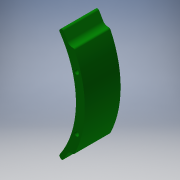
# Autodesk Inventor part: Goal
Saved by Autodesk Inventor 2016 (Build 200138000, 138)
## iProperties
Created: 2015-08-20
Part Number: Goal
Material: Generic
Document SubType Name: Modeling
Designer: TFHulbert
Density: 1 g/cm^3
Appearance: Default
Author: TFHulbert
Autodesk Inventor part; units mm, degrees
ref_plane "XZ Plane" through (0, 0, 0) normal (0, 1, 0) x (-1, 0, 0)
ref_plane "XY Plane" through (0, 0, 0) normal (0, 0, 1) x (1, 0, 0)
sketch "Sketch2" plane through (0, 0, 0) normal (0, 1, 0) x (-1, 0, 0)
  arc A0 (-3.565, 94.6695) -> (-3.565, -8.3744) centre (100.201, 43.1475) ccw
  arc A1 (10.972, -26.9746) -> (17.7694, -18.565) centre (-67.181, 43.1475) ccw
  arc A2 (17.7694, -18.565) -> (17.7741, -16.2207) centre (16.1512, -17.3895) ccw
  arc A3 (17.7741, 102.5157) -> (17.7741, -16.2207) centre (100.201, 43.1475) ccw
  arc A4 (17.7741, 102.5157) -> (17.7694, 104.8601) centre (16.1512, 103.6846) ccw
  arc A5 (17.7694, 104.8601) -> (10.972, 113.2697) centre (-67.181, 43.1475) ccw
  arc A6 (-3.565, 94.6695) -> (3.8676, 97.5325) centre (-1.6208, 100.7012) ccw
  line L0 (3.8676, 97.5325) -> (9.8686, 107.9266)
  arc A7 (13.2665, 103.6551) -> (9.8686, 107.9266) centre (-67.181, 43.1475) ccw
  arc A8 (13.2665, 103.6551) -> (13.2665, -17.36) centre (100.201, 43.1475) ccw
  arc A9 (9.8686, -21.6316) -> (13.2665, -17.36) centre (-67.181, 43.1475) ccw
  line L1 (9.8686, -21.6316) -> (3.8676, -11.2375)
  arc A10 (3.8676, -11.2375) -> (-3.565, -8.3744) centre (-1.6208, -14.4061) ccw
  line L2 (-6.3804, 13.1475) -> (-1.3804, 13.1475)
  line L3 (17.3738, -14.7626) -> (18.7645, -17.1714)
  circle A11 centre (-6.3804, 73.1475) radius 2.5
  circle A12 centre (-6.3804, 13.1475) radius 2.5
  arc A13 (-2.6208, 98.9692) -> (-1.4601, 98.7077) centre (-1.6208, 100.7012) ccw
  point P0 (0, 0)
  constraints: 25 point on circle, 14 centre point, 8 end point
extrude "Extrusion2" add sketch "Sketch2" along normal blind 40
fillet "Fillet4" radius 2 6 edges at (-9.8686, 20, 107.9266) (3.565, 20, 94.6695) (-13.2665, 20, 103.6551) (-13.2665, 20, -17.36) (-9.8686, 20, -21.6316) (3.565, 20, -8.3744)
ref_plane "Work Plane1" through (-13.25, 0, 0) normal (-1, 0, 0) x (0, -1, 0)
sketch "Sketch4" plane through (-13.25, 0, 0) normal (-1, 0, 0) x (0, -1, 0)
  line L0 (-31.9197, 26.5555) -> (-31.9197, 59.312) construction
  line L1 (-31.9197, 59.312) -> (-10.9843, 59.312) construction
  line L2 (-10.9843, 59.312) -> (-10.9843, 26.5555) construction
  line L3 (-10.9843, 26.5555) -> (-31.9197, 26.5555) construction
  line L4 (0, -20.122) -> (-40, -20.122) projected
  line L5 (-40, 105.4171) -> (-40, 106.4171) projected
  line L6 (-40, -20.122) -> (-40, 106.4171)
  line L7 (-40, -16.1771) -> (-40, 102.4722) projected
  line L8 (-40, 43.1475) -> (-4.7304, 43.1475)
  spline S0 degree 2 poles (-29.9161, 28.2102) (-29.9161, 27.8593) (-30.0521, 27.3303) (-30.1509, 27.1029) knots 0 0 0 1 2 2 2
  line L9 (-30.1509, 27.1029) -> (-30.8776, 27.1029)
  line L10 (-30.8776, 27.1029) -> (-30.8776, 27.1721)
  spline S1 degree 2 poles (-30.8776, 27.1721) (-30.6823, 27.402) (-30.4723, 27.9532) (-30.4723, 28.2127) knots 0 0 0 1 2 2 2
  spline S2 degree 2 poles (-30.4723, 28.2127) (-30.4723, 28.2794) (-30.5019, 28.4945) (-30.5316, 28.5587) knots 0 0 0 1 2 2 2
  spline S3 degree 2 poles (-30.5316, 28.5587) (-30.5662, 28.6378) (-30.6922, 28.7491) (-30.7936, 28.7491) knots 0 0 0 1 2 2 2
  spline S4 degree 2 poles (-30.7936, 28.7491) (-30.9097, 28.7491) (-31.0531, 28.5686) (-31.0852, 28.445) knots 0 0 0 1 2 2 2
  spline S5 degree 2 poles (-31.0852, 28.445) (-31.1272, 28.2893) (-31.1989, 27.9359) (-31.2533, 27.7802) knots 0 0 0 1 2 2 2
  spline S6 degree 2 poles (-31.2533, 27.7802) (-31.3769, 27.4267) (-31.7995, 27.1202) (-32.1159, 27.1202) knots 0 0 0 1 2 2 2
  spline S7 degree 2 poles (-32.1159, 27.1202) (-32.5435, 27.1202) (-33.0749, 27.8444) (-33.0749, 28.3882) knots 0 0 0 1 2 2 2
  spline S8 degree 2 poles (-33.0749, 28.3882) (-33.0749, 28.6601) (-32.9637, 29.1989) (-32.8697, 29.4115) knots 0 0 0 1 2 2 2
  line L11 (-32.8697, 29.4115) -> (-32.1727, 29.4115)
  line L12 (-32.1727, 29.4115) -> (-32.1727, 29.3447)
  spline S9 degree 2 poles (-32.1727, 29.3447) (-32.3186, 29.1742) (-32.5188, 28.6848) (-32.5188, 28.4277) knots 0 0 0 1 2 2 2
  spline S10 degree 2 poles (-32.5188, 28.4277) (-32.5188, 28.3264) (-32.4891, 28.1682) (-32.4496, 28.0792) knots 0 0 0 1 2 2 2
  spline S11 degree 2 poles (-32.4496, 28.0792) (-32.4174, 28.0076) (-32.2889, 27.9038) (-32.2098, 27.9038) knots 0 0 0 1 2 2 2
  spline S12 degree 2 poles (-32.2098, 27.9038) (-32.0912, 27.9038) (-31.9552, 28.0694) (-31.9009, 28.3066) knots 0 0 0 1 2 2 2
  spline S13 degree 2 poles (-31.9009, 28.3066) (-31.8663, 28.4599) (-31.7995, 28.7441) (-31.7427, 28.9072) knots 0 0 0 1 2 2 2
  spline S14 degree 2 poles (-31.7427, 28.9072) (-31.6265, 29.2236) (-31.2409, 29.5326) (-30.9246, 29.5326) knots 0 0 0 1 2 2 2
  spline S15 degree 2 poles (-30.9246, 29.5326) (-30.4698, 29.5326) (-29.9161, 28.8183) (-29.9161, 28.2102) knots 0 0 0 1 2 2 2
  line L13 (-29.9705, 32.4985) -> (-29.9705, 31.7323)
  line L14 (-29.9705, 31.7323) -> (-31.3225, 31.7323)
  line L15 (-31.3225, 31.7323) -> (-31.3225, 30.6918)
  line L16 (-31.3225, 30.6918) -> (-29.9705, 30.6918)
  line L17 (-29.9705, 30.6918) -> (-29.9705, 29.9256)
  line L18 (-29.9705, 29.9256) -> (-33.0205, 29.9256)
  line L19 (-33.0205, 29.9256) -> (-33.0205, 30.6918)
  line L20 (-33.0205, 30.6918) -> (-31.9033, 30.6918)
  line L21 (-31.9033, 30.6918) -> (-31.9033, 31.7323)
  line L22 (-31.9033, 31.7323) -> (-33.0205, 31.7323)
  line L23 (-33.0205, 31.7323) -> (-33.0205, 32.4985)
  line L24 (-33.0205, 32.4985) -> (-29.9705, 32.4985)
  line L25 (-32.4397, 35.1728) -> (-32.4397, 33.8925)
  line L26 (-32.4397, 33.8925) -> (-31.8638, 33.8925)
  line L27 (-31.8638, 33.8925) -> (-31.8638, 35.0715)
  line L28 (-31.8638, 35.0715) -> (-31.2829, 35.0715)
  line L29 (-31.2829, 35.0715) -> (-31.2829, 33.8925)
  line L30 (-31.2829, 33.8925) -> (-29.9705, 33.8925)
  line L31 (-29.9705, 33.8925) -> (-29.9705, 33.1313)
  line L32 (-29.9705, 33.1313) -> (-33.0205, 33.1313)
  line L33 (-33.0205, 33.1313) -> (-33.0205, 35.1728)
  line L34 (-33.0205, 35.1728) -> (-32.4397, 35.1728)
  line L35 (-29.9705, 39.6144) -> (-29.9705, 38.6826)
  line L36 (-29.9705, 38.6826) -> (-31.0902, 37.8348)
  line L37 (-31.0902, 37.8348) -> (-31.0902, 37.558)
  line L38 (-31.0902, 37.558) -> (-29.9705, 37.558)
  line L39 (-29.9705, 37.558) -> (-29.9705, 36.7967)
  line L40 (-29.9705, 36.7967) -> (-33.0205, 36.7967)
  line L41 (-33.0205, 36.7967) -> (-33.0205, 38.0226)
  spline S16 degree 2 poles (-33.0205, 38.0226) (-33.0205, 38.2772) (-32.9562, 38.6529) (-32.8574, 38.8136) knots 0 0 0 1 2 2 2
  spline S17 degree 2 poles (-32.8574, 38.8136) (-32.7536, 38.9767) (-32.4298, 39.1695) (-32.1826, 39.1695) knots 0 0 0 1 2 2 2
  spline S18 degree 2 poles (-32.1826, 39.1695) (-31.8341, 39.1695) (-31.3966, 38.8531) (-31.2681, 38.5886) knots 0 0 0 1 2 2 2
  line L42 (-31.2681, 38.5886) -> (-29.9705, 39.6144)
  spline S19 degree 2 poles (-32.0862, 38.3835) (-32.2024, 38.3835) (-32.368, 38.2945) (-32.4125, 38.1932) knots 0 0 0 1 2 2 2
  spline S20 degree 2 poles (-32.4125, 38.1932) (-32.4421, 38.1215) (-32.4594, 37.946) (-32.4594, 37.815) knots 0 0 0 1 2 2 2
  line L43 (-32.4594, 37.815) -> (-32.4594, 37.558)
  line L44 (-32.4594, 37.558) -> (-31.6389, 37.558)
  line L45 (-31.6389, 37.558) -> (-31.6389, 37.7779)
  spline S21 degree 2 poles (-31.6389, 37.7779) (-31.6389, 37.9361) (-31.6784, 38.161) (-31.7402, 38.2377) knots 0 0 0 1 2 2 2
  spline S22 degree 2 poles (-31.7402, 38.2377) (-31.7995, 38.3118) (-31.9577, 38.3835) (-32.0862, 38.3835) knots 0 0 0 1 2 2 2
  spline S23 degree 2 poles (-31.4955, 42.6174) (-30.754, 42.6174) (-29.9062, 41.8265) (-29.9062, 41.1394) knots 0 0 0 1 2 2 2
  spline S24 degree 2 poles (-29.9062, 41.1394) (-29.9062, 40.4498) (-30.7639, 39.6638) (-31.4955, 39.6638) knots 0 0 0 1 2 2 2
  spline S25 degree 2 poles (-31.4955, 39.6638) (-32.2296, 39.6638) (-33.0848, 40.4498) (-33.0848, 41.1394) knots 0 0 0 1 2 2 2
  spline S26 degree 2 poles (-33.0848, 41.1394) (-33.0848, 41.8265) (-32.2345, 42.6174) (-31.4955, 42.6174) knots 0 0 0 1 2 2 2
  spline S27 degree 2 poles (-31.4955, 41.8265) (-31.7699, 41.8265) (-32.153, 41.7153) (-32.2741, 41.6189) knots 0 0 0 1 2 2 2
  spline S28 degree 2 poles (-32.2741, 41.6189) (-32.4001, 41.5225) (-32.5089, 41.2753) (-32.5089, 41.1418) knots 0 0 0 1 2 2 2
  spline S29 degree 2 poles (-32.5089, 41.1418) (-32.5089, 41.001) (-32.4075, 40.7711) (-32.279, 40.6648) knots 0 0 0 1 2 2 2
  spline S30 degree 2 poles (-32.279, 40.6648) (-32.1604, 40.5709) (-31.7674, 40.4547) (-31.4955, 40.4547) knots 0 0 0 1 2 2 2
  spline S31 degree 2 poles (-31.4955, 40.4547) (-31.2137, 40.4547) (-30.843, 40.5659) (-30.7169, 40.6623) knots 0 0 0 1 2 2 2
  spline S32 degree 2 poles (-30.7169, 40.6623) (-30.5909, 40.7587) (-30.4821, 41.0084) (-30.4821, 41.1418) knots 0 0 0 1 2 2 2
  spline S33 degree 2 poles (-30.4821, 41.1418) (-30.4821, 41.2778) (-30.5983, 41.5299) (-30.7219, 41.6213) knots 0 0 0 1 2 2 2
  spline S34 degree 2 poles (-30.7219, 41.6213) (-30.8554, 41.7202) (-31.2088, 41.8265) (-31.4955, 41.8265) knots 0 0 0 1 2 2 2
  spline S35 degree 2 poles (-30.9048, 45.5092) (-30.6774, 45.5092) (-30.3338, 45.3362) (-30.2201, 45.1929) knots 0 0 0 1 2 2 2
  spline S36 degree 2 poles (-30.2201, 45.1929) (-30.0842, 45.0198) (-29.9705, 44.6095) (-29.9705, 44.2907) knots 0 0 0 1 2 2 2
  line L46 (-29.9705, 44.2907) -> (-29.9705, 43.0722)
  line L47 (-29.9705, 43.0722) -> (-33.0205, 43.0722)
  line L48 (-33.0205, 43.0722) -> (-33.0205, 44.1474)
  spline S37 degree 2 poles (-33.0205, 44.1474) (-33.0205, 44.4835) (-32.9686, 44.8295) (-32.887, 44.9803) knots 0 0 0 1 2 2 2
  spline S38 degree 2 poles (-32.887, 44.9803) (-32.8005, 45.1459) (-32.5039, 45.3065) (-32.3111, 45.3065) knots 0 0 0 1 2 2 2
  spline S39 degree 2 poles (-32.3111, 45.3065) (-32.0887, 45.3065) (-31.7402, 45.0841) (-31.6586, 44.8864) knots 0 0 0 1 2 2 2
  line L49 (-31.6586, 44.8864) -> (-31.6438, 44.8864)
  spline S40 degree 2 poles (-31.6438, 44.8864) (-31.5845, 45.1706) (-31.2162, 45.5092) (-30.9048, 45.5092) knots 0 0 0 1 2 2 2
  spline S41 degree 2 poles (-30.9171, 44.7183) (-31.0605, 44.7183) (-31.2212, 44.6046) (-31.2632, 44.4909) knots 0 0 0 1 2 2 2
  spline S42 degree 2 poles (-31.2632, 44.4909) (-31.2904, 44.4217) (-31.2953, 44.177) (-31.2953, 43.9743) knots 0 0 0 1 2 2 2
  line L50 (-31.2953, 43.9743) -> (-31.2953, 43.8335)
  line L51 (-31.2953, 43.8335) -> (-30.5266, 43.8335)
  line L52 (-30.5266, 43.8335) -> (-30.5266, 43.8755)
  spline S43 degree 2 poles (-30.5266, 43.8755) (-30.5266, 44.1721) (-30.534, 44.3995) (-30.5859, 44.5181) knots 0 0 0 1 2 2 2
  spline S44 degree 2 poles (-30.5859, 44.5181) (-30.6329, 44.6219) (-30.8059, 44.7183) (-30.9171, 44.7183) knots 0 0 0 1 2 2 2
  spline S45 degree 2 poles (-32.1604, 44.528) (-32.2345, 44.528) (-32.3902, 44.4514) (-32.4248, 44.3723) knots 0 0 0 1 2 2 2
  spline S46 degree 2 poles (-32.4248, 44.3723) (-32.4594, 44.2981) (-32.4644, 44.0905) (-32.4644, 43.8854) knots 0 0 0 1 2 2 2
  line L53 (-32.4644, 43.8854) -> (-32.4644, 43.8335)
  line L54 (-32.4644, 43.8335) -> (-31.8168, 43.8335)
  line L55 (-31.8168, 43.8335) -> (-31.8168, 43.9298)
  spline S47 degree 2 poles (-31.8168, 43.9298) (-31.8168, 44.1251) (-31.8242, 44.2833) (-31.8638, 44.3673) knots 0 0 0 1 2 2 2
  spline S48 degree 2 poles (-31.8638, 44.3673) (-31.9083, 44.4588) (-32.059, 44.528) (-32.1604, 44.528) knots 0 0 0 1 2 2 2
  spline S49 degree 2 poles (-31.4955, 48.7248) (-30.754, 48.7248) (-29.9062, 47.9339) (-29.9062, 47.2468) knots 0 0 0 1 2 2 2
  spline S50 degree 2 poles (-29.9062, 47.2468) (-29.9062, 46.5572) (-30.7639, 45.7712) (-31.4955, 45.7712) knots 0 0 0 1 2 2 2
  spline S51 degree 2 poles (-31.4955, 45.7712) (-32.2296, 45.7712) (-33.0848, 46.5572) (-33.0848, 47.2468) knots 0 0 0 1 2 2 2
  spline S52 degree 2 poles (-33.0848, 47.2468) (-33.0848, 47.9339) (-32.2345, 48.7248) (-31.4955, 48.7248) knots 0 0 0 1 2 2 2
  spline S53 degree 2 poles (-31.4955, 47.9339) (-31.7699, 47.9339) (-32.153, 47.8227) (-32.2741, 47.7263) knots 0 0 0 1 2 2 2
  spline S54 degree 2 poles (-32.2741, 47.7263) (-32.4001, 47.6299) (-32.5089, 47.3827) (-32.5089, 47.2493) knots 0 0 0 1 2 2 2
  spline S55 degree 2 poles (-32.5089, 47.2493) (-32.5089, 47.1084) (-32.4075, 46.8785) (-32.279, 46.7722) knots 0 0 0 1 2 2 2
  spline S56 degree 2 poles (-32.279, 46.7722) (-32.1604, 46.6783) (-31.7674, 46.5621) (-31.4955, 46.5621) knots 0 0 0 1 2 2 2
  spline S57 degree 2 poles (-31.4955, 46.5621) (-31.2137, 46.5621) (-30.843, 46.6734) (-30.7169, 46.7698) knots 0 0 0 1 2 2 2
  spline S58 degree 2 poles (-30.7169, 46.7698) (-30.5909, 46.8662) (-30.4821, 47.1158) (-30.4821, 47.2493) knots 0 0 0 1 2 2 2
  spline S59 degree 2 poles (-30.4821, 47.2493) (-30.4821, 47.3852) (-30.5983, 47.6373) (-30.7219, 47.7288) knots 0 0 0 1 2 2 2
  spline S60 degree 2 poles (-30.7219, 47.7288) (-30.8554, 47.8276) (-31.2088, 47.9339) (-31.4955, 47.9339) knots 0 0 0 1 2 2 2
  line L56 (-29.9705, 49.7654) -> (-32.4397, 49.7654)
  line L57 (-32.4397, 49.7654) -> (-32.4397, 48.8632)
  line L58 (-32.4397, 48.8632) -> (-33.0205, 48.8632)
  line L59 (-33.0205, 48.8632) -> (-33.0205, 51.4337)
  line L60 (-33.0205, 51.4337) -> (-32.4397, 51.4337)
  line L61 (-32.4397, 51.4337) -> (-32.4397, 50.5316)
  line L62 (-32.4397, 50.5316) -> (-29.9705, 50.5316)
  line L63 (-29.9705, 50.5316) -> (-29.9705, 49.7654)
  line L64 (-29.9705, 53.2652) -> (-29.9705, 51.6241)
  line L65 (-29.9705, 51.6241) -> (-30.5019, 51.6241)
  line L66 (-30.5019, 51.6241) -> (-30.5019, 52.0615)
  line L67 (-30.5019, 52.0615) -> (-32.4891, 52.0615)
  line L68 (-32.4891, 52.0615) -> (-32.4891, 51.6241)
  line L69 (-32.4891, 51.6241) -> (-33.0205, 51.6241)
  line L70 (-33.0205, 51.6241) -> (-33.0205, 53.2652)
  line L71 (-33.0205, 53.2652) -> (-32.4891, 53.2652)
  line L72 (-32.4891, 53.2652) -> (-32.4891, 52.8277)
  line L73 (-32.4891, 52.8277) -> (-30.5019, 52.8277)
  line L74 (-30.5019, 52.8277) -> (-30.5019, 53.2652)
  line L75 (-30.5019, 53.2652) -> (-29.9705, 53.2652)
  spline S61 degree 2 poles (-29.9112, 55.0893) (-29.9112, 54.4022) (-30.7417, 53.5964) (-31.493, 53.5964) knots 0 0 0 1 2 2 2
  spline S62 degree 2 poles (-31.493, 53.5964) (-32.2172, 53.5964) (-33.0798, 54.4046) (-33.0798, 55.0918) knots 0 0 0 1 2 2 2
  spline S63 degree 2 poles (-33.0798, 55.0918) (-33.0798, 55.2722) (-33.0378, 55.5638) (-33.0032, 55.6973) knots 0 0 0 1 2 2 2
  spline S64 degree 2 poles (-33.0032, 55.6973) (-32.9711, 55.8011) (-32.8648, 56.0458) (-32.8252, 56.1224) knots 0 0 0 1 2 2 2
  line L76 (-32.8252, 56.1224) -> (-32.0986, 56.1224)
  line L77 (-32.0986, 56.1224) -> (-32.0986, 56.0458)
  spline S65 degree 2 poles (-32.0986, 56.0458) (-32.148, 55.989) (-32.2864, 55.8209) (-32.3507, 55.7146) knots 0 0 0 1 2 2 2
  spline S66 degree 2 poles (-32.3507, 55.7146) (-32.4174, 55.6083) (-32.5089, 55.3538) (-32.5089, 55.2129) knots 0 0 0 1 2 2 2
  spline S67 degree 2 poles (-32.5089, 55.2129) (-32.5089, 55.0473) (-32.4051, 54.7729) (-32.2741, 54.6469) knots 0 0 0 1 2 2 2
  spline S68 degree 2 poles (-32.2741, 54.6469) (-32.1579, 54.5332) (-31.76, 54.3873) (-31.4906, 54.3873) knots 0 0 0 1 2 2 2
  spline S69 degree 2 poles (-31.4906, 54.3873) (-31.2063, 54.3873) (-30.8183, 54.5381) (-30.6996, 54.6617) knots 0 0 0 1 2 2 2
  spline S70 degree 2 poles (-30.6996, 54.6617) (-30.5835, 54.7803) (-30.4821, 55.072) (-30.4821, 55.2178) knots 0 0 0 1 2 2 2
  spline S71 degree 2 poles (-30.4821, 55.2178) (-30.4821, 55.3686) (-30.5835, 55.6429) (-30.6453, 55.7369) knots 0 0 0 1 2 2 2
  spline S72 degree 2 poles (-30.6453, 55.7369) (-30.7071, 55.8407) (-30.8381, 55.9964) (-30.89, 56.0532) knots 0 0 0 1 2 2 2
  line L78 (-30.89, 56.0532) -> (-30.89, 56.1224)
  line L79 (-30.89, 56.1224) -> (-30.1732, 56.1224)
  spline S73 degree 2 poles (-30.1732, 56.1224) (-30.1336, 56.0384) (-30.0348, 55.8184) (-30.0002, 55.6998) knots 0 0 0 1 2 2 2
  spline S74 degree 2 poles (-30.0002, 55.6998) (-29.9557, 55.5564) (-29.9112, 55.3068) (-29.9112, 55.0893) knots 0 0 0 1 2 2 2
  spline S75 degree 2 poles (-29.9161, 57.5164) (-29.9161, 57.1655) (-30.0521, 56.6365) (-30.1509, 56.4091) knots 0 0 0 1 2 2 2
  line L80 (-30.1509, 56.4091) -> (-30.8776, 56.4091)
  line L81 (-30.8776, 56.4091) -> (-30.8776, 56.4783)
  spline S76 degree 2 poles (-30.8776, 56.4783) (-30.6823, 56.7082) (-30.4723, 57.2594) (-30.4723, 57.5189) knots 0 0 0 1 2 2 2
  spline S77 degree 2 poles (-30.4723, 57.5189) (-30.4723, 57.5856) (-30.5019, 57.8007) (-30.5316, 57.8649) knots 0 0 0 1 2 2 2
  spline S78 degree 2 poles (-30.5316, 57.8649) (-30.5662, 57.944) (-30.6922, 58.0553) (-30.7936, 58.0553) knots 0 0 0 1 2 2 2
  spline S79 degree 2 poles (-30.7936, 58.0553) (-30.9097, 58.0553) (-31.0531, 57.8748) (-31.0852, 57.7512) knots 0 0 0 1 2 2 2
  spline S80 degree 2 poles (-31.0852, 57.7512) (-31.1272, 57.5955) (-31.1989, 57.2421) (-31.2533, 57.0864) knots 0 0 0 1 2 2 2
  spline S81 degree 2 poles (-31.2533, 57.0864) (-31.3769, 56.7329) (-31.7995, 56.4264) (-32.1159, 56.4264) knots 0 0 0 1 2 2 2
  spline S82 degree 2 poles (-32.1159, 56.4264) (-32.5435, 56.4264) (-33.0749, 57.1506) (-33.0749, 57.6944) knots 0 0 0 1 2 2 2
  spline S83 degree 2 poles (-33.0749, 57.6944) (-33.0749, 57.9663) (-32.9637, 58.5051) (-32.8697, 58.7177) knots 0 0 0 1 2 2 2
  line L82 (-32.8697, 58.7177) -> (-32.1727, 58.7177)
  line L83 (-32.1727, 58.7177) -> (-32.1727, 58.6509)
  spline S84 degree 2 poles (-32.1727, 58.6509) (-32.3186, 58.4804) (-32.5188, 57.991) (-32.5188, 57.7339) knots 0 0 0 1 2 2 2
  spline S85 degree 2 poles (-32.5188, 57.7339) (-32.5188, 57.6326) (-32.4891, 57.4744) (-32.4496, 57.3854) knots 0 0 0 1 2 2 2
  spline S86 degree 2 poles (-32.4496, 57.3854) (-32.4174, 57.3138) (-32.2889, 57.21) (-32.2098, 57.21) knots 0 0 0 1 2 2 2
  spline S87 degree 2 poles (-32.2098, 57.21) (-32.0912, 57.21) (-31.9552, 57.3756) (-31.9009, 57.6128) knots 0 0 0 1 2 2 2
  spline S88 degree 2 poles (-31.9009, 57.6128) (-31.8663, 57.7661) (-31.7995, 58.0503) (-31.7427, 58.2134) knots 0 0 0 1 2 2 2
  spline S89 degree 2 poles (-31.7427, 58.2134) (-31.6265, 58.5298) (-31.2409, 58.8388) (-30.9246, 58.8388) knots 0 0 0 1 2 2 2
  spline S90 degree 2 poles (-30.9246, 58.8388) (-30.4698, 58.8388) (-29.9161, 58.1245) (-29.9161, 57.5164) knots 0 0 0 1 2 2 2
  line L84 (-24.9488, 40.1408) -> (-24.9488, 37.8991)
  line L85 (-24.9488, 37.8991) -> (-25.4456, 37.8991)
  spline S91 degree 2 poles (-25.4456, 37.8991) (-25.673, 38.1833) (-26.0734, 38.6381) (-26.2538, 38.8086) knots 0 0 0 1 2 2 2
  spline S92 degree 2 poles (-26.2538, 38.8086) (-26.4886, 39.0335) (-26.847, 39.2337) (-27.0348, 39.2337) knots 0 0 0 1 2 2 2
  spline S93 degree 2 poles (-27.0348, 39.2337) (-27.2474, 39.2337) (-27.4748, 38.9792) (-27.4748, 38.7518) knots 0 0 0 1 2 2 2
  spline S94 degree 2 poles (-27.4748, 38.7518) (-27.4748, 38.6356) (-27.4179, 38.428) (-27.3734, 38.3217) knots 0 0 0 1 2 2 2
  spline S95 degree 2 poles (-27.3734, 38.3217) (-27.3265, 38.2179) (-27.2276, 38.0696) (-27.2029, 38.0325) knots 0 0 0 1 2 2 2
  line L86 (-27.2029, 38.0325) -> (-27.2029, 37.9732)
  line L87 (-27.2029, 37.9732) -> (-27.8678, 37.9732)
  spline S96 degree 2 poles (-27.8678, 37.9732) (-27.9296, 38.1017) (-28.0581, 38.6504) (-28.0581, 38.905) knots 0 0 0 1 2 2 2
  spline S97 degree 2 poles (-28.0581, 38.905) (-28.0581, 39.4488) (-27.5736, 40.0074) (-27.1362, 40.0074) knots 0 0 0 1 2 2 2
  spline S98 degree 2 poles (-27.1362, 40.0074) (-26.8668, 40.0074) (-26.3477, 39.7528) (-26.0511, 39.4587) knots 0 0 0 1 2 2 2
  spline S99 degree 2 poles (-26.0511, 39.4587) (-25.8682, 39.2733) (-25.584, 38.9248) (-25.5247, 38.8482) knots 0 0 0 1 2 2 2
  line L88 (-25.5247, 38.8482) -> (-25.5247, 40.1408)
  line L89 (-25.5247, 40.1408) -> (-24.9488, 40.1408)
  spline S100 degree 2 poles (-26.4738, 42.7731) (-26.0783, 42.7731) (-25.4851, 42.6471) (-25.2849, 42.5062) knots 0 0 0 1 2 2 2
  spline S101 degree 2 poles (-25.2849, 42.5062) (-25.0872, 42.3678) (-24.8845, 41.9204) (-24.8845, 41.5991) knots 0 0 0 1 2 2 2
  spline S102 degree 2 poles (-24.8845, 41.5991) (-24.8845, 41.2753) (-25.0872, 40.8304) (-25.2898, 40.6895) knots 0 0 0 1 2 2 2
  spline S103 degree 2 poles (-25.2898, 40.6895) (-25.4901, 40.5486) (-26.0783, 40.4226) (-26.4738, 40.4226) knots 0 0 0 1 2 2 2
  spline S104 degree 2 poles (-26.4738, 40.4226) (-26.8791, 40.4226) (-27.4525, 40.5486) (-27.6601, 40.692) knots 0 0 0 1 2 2 2
  spline S105 degree 2 poles (-27.6601, 40.692) (-27.8628, 40.8354) (-28.0606, 41.2877) (-28.0606, 41.5991) knots 0 0 0 1 2 2 2
  spline S106 degree 2 poles (-28.0606, 41.5991) (-28.0606, 41.9278) (-27.8529, 42.3678) (-27.6478, 42.5087) knots 0 0 0 1 2 2 2
  spline S107 degree 2 poles (-27.6478, 42.5087) (-27.4476, 42.6471) (-26.8569, 42.7731) (-26.4738, 42.7731) knots 0 0 0 1 2 2 2
  spline S108 degree 2 poles (-26.4738, 42.0044) (-27.0398, 42.0044) (-27.497, 41.8191) (-27.497, 41.5991) knots 0 0 0 1 2 2 2
  spline S109 degree 2 poles (-27.497, 41.5991) (-27.497, 41.3791) (-27.0398, 41.1913) (-26.4713, 41.1913) knots 0 0 0 1 2 2 2
  spline S110 degree 2 poles (-26.4713, 41.1913) (-25.9127, 41.1913) (-25.448, 41.3791) (-25.448, 41.5991) knots 0 0 0 1 2 2 2
  spline S111 degree 2 poles (-25.448, 41.5991) (-25.448, 41.8166) (-25.9127, 42.0044) (-26.4738, 42.0044) knots 0 0 0 1 2 2 2
  line L90 (-24.9488, 45.3486) -> (-24.9488, 43.3342)
  line L91 (-24.9488, 43.3342) -> (-25.4802, 43.3342)
  line L92 (-25.4802, 43.3342) -> (-25.4802, 43.9768)
  line L93 (-25.4802, 43.9768) -> (-27.0941, 43.9768)
  line L94 (-27.0941, 43.9768) -> (-27.0941, 43.3342)
  line L95 (-27.0941, 43.3342) -> (-27.5909, 43.3342)
  spline S112 degree 2 poles (-27.5909, 43.3342) (-27.5909, 43.4751) (-27.628, 43.7544) (-27.6676, 43.8384) knots 0 0 0 1 2 2 2
  spline S113 degree 2 poles (-27.6676, 43.8384) (-27.717, 43.9348) (-27.8826, 44.0435) (-28.0062, 44.0534) knots 0 0 0 1 2 2 2
  line L96 (-28.0062, 44.0534) -> (-28.0062, 44.7208)
  line L97 (-28.0062, 44.7208) -> (-25.4802, 44.7208)
  line L98 (-25.4802, 44.7208) -> (-25.4802, 45.3486)
  line L99 (-25.4802, 45.3486) -> (-24.9488, 45.3486)
  spline S114 degree 2 poles (-25.9819, 48.0871) (-25.7422, 48.0871) (-25.3368, 47.924) (-25.191, 47.7634) knots 0 0 0 1 2 2 2
  spline S115 degree 2 poles (-25.191, 47.7634) (-25.0452, 47.6027) (-24.8845, 47.1627) (-24.8845, 46.8414) knots 0 0 0 1 2 2 2
  spline S116 degree 2 poles (-24.8845, 46.8414) (-24.887, 46.5003) (-24.9982, 46.011) (-25.0699, 45.8503) knots 0 0 0 1 2 2 2
  line L100 (-25.0699, 45.8503) -> (-25.7347, 45.8503)
  line L101 (-25.7347, 45.8503) -> (-25.7347, 45.9195)
  spline S117 degree 2 poles (-25.7347, 45.9195) (-25.7026, 45.9788) (-25.6186, 46.1222) (-25.5741, 46.2384) knots 0 0 0 1 2 2 2
  spline S118 degree 2 poles (-25.5741, 46.2384) (-25.5321, 46.3471) (-25.4752, 46.572) (-25.4752, 46.708) knots 0 0 0 1 2 2 2
  spline S119 degree 2 poles (-25.4752, 46.708) (-25.4752, 46.8266) (-25.5345, 47.1034) (-25.6136, 47.1875) knots 0 0 0 1 2 2 2
  spline S120 degree 2 poles (-25.6136, 47.1875) (-25.6754, 47.2493) (-25.8262, 47.3185) (-25.9522, 47.3185) knots 0 0 0 1 2 2 2
  spline S121 degree 2 poles (-25.9522, 47.3185) (-26.061, 47.3185) (-26.2142, 47.2295) (-26.2612, 47.1578) knots 0 0 0 1 2 2 2
  spline S122 degree 2 poles (-26.2612, 47.1578) (-26.3304, 47.054) (-26.37, 46.7574) (-26.37, 46.6511) knots 0 0 0 1 2 2 2
  spline S123 degree 2 poles (-26.37, 46.6511) (-26.37, 46.483) (-26.3156, 46.1642) (-26.2859, 46.048) knots 0 0 0 1 2 2 2
  line L102 (-26.2859, 46.048) -> (-26.2859, 45.9813)
  line L103 (-26.2859, 45.9813) -> (-27.9988, 45.9813)
  line L104 (-27.9988, 45.9813) -> (-27.9988, 48.0031)
  line L105 (-27.9988, 48.0031) -> (-27.4229, 48.0031)
  line L106 (-27.4229, 48.0031) -> (-27.4229, 46.7055)
  line L107 (-27.4229, 46.7055) -> (-26.9162, 46.7055)
  spline S124 degree 2 poles (-26.9162, 46.7055) (-26.9211, 46.7673) (-26.9261, 46.9378) (-26.9261, 46.9848) knots 0 0 0 1 2 2 2
  spline S125 degree 2 poles (-26.9261, 46.9848) (-26.9261, 47.2048) (-26.8371, 47.5755) (-26.7456, 47.7213) knots 0 0 0 1 2 2 2
  spline S126 degree 2 poles (-26.7456, 47.7213) (-26.6319, 47.8944) (-26.2538, 48.0871) (-25.9819, 48.0871) knots 0 0 0 1 2 2 2
  line L108 (-19.927, 33.6194) -> (-22.3962, 33.6194)
  line L109 (-22.3962, 33.6194) -> (-22.3962, 32.7173)
  line L110 (-22.3962, 32.7173) -> (-22.977, 32.7173)
  line L111 (-22.977, 32.7173) -> (-22.977, 35.2878)
  line L112 (-22.977, 35.2878) -> (-22.3962, 35.2878)
  line L113 (-22.3962, 35.2878) -> (-22.3962, 34.3856)
  line L114 (-22.3962, 34.3856) -> (-19.927, 34.3856)
  line L115 (-19.927, 34.3856) -> (-19.927, 33.6194)
  line L116 (-22.3962, 38.8716) -> (-22.3962, 37.5913)
  line L117 (-22.3962, 37.5913) -> (-21.8203, 37.5913)
  line L118 (-21.8203, 37.5913) -> (-21.8203, 38.7703)
  line L119 (-21.8203, 38.7703) -> (-21.2395, 38.7703)
  line L120 (-21.2395, 38.7703) -> (-21.2395, 37.5913)
  line L121 (-21.2395, 37.5913) -> (-19.927, 37.5913)
  line L122 (-19.927, 37.5913) -> (-19.927, 36.8301)
  line L123 (-19.927, 36.8301) -> (-22.977, 36.8301)
  line L124 (-22.977, 36.8301) -> (-22.977, 38.8716)
  line L125 (-22.977, 38.8716) -> (-22.3962, 38.8716)
  line L126 (-19.927, 42.0848) -> (-19.927, 41.153)
  line L127 (-19.927, 41.153) -> (-21.0467, 40.3052)
  line L128 (-21.0467, 40.3052) -> (-21.0467, 40.0284)
  line L129 (-21.0467, 40.0284) -> (-19.927, 40.0284)
  line L130 (-19.927, 40.0284) -> (-19.927, 39.2671)
  line L131 (-19.927, 39.2671) -> (-22.977, 39.2671)
  line L132 (-22.977, 39.2671) -> (-22.977, 40.493)
  spline S127 degree 2 poles (-22.977, 40.493) (-22.977, 40.7476) (-22.9128, 41.1233) (-22.8139, 41.284) knots 0 0 0 1 2 2 2
  spline S128 degree 2 poles (-22.8139, 41.284) (-22.7101, 41.4471) (-22.3863, 41.6399) (-22.1391, 41.6399) knots 0 0 0 1 2 2 2
  spline S129 degree 2 poles (-22.1391, 41.6399) (-21.7906, 41.6399) (-21.3532, 41.3235) (-21.2246, 41.059) knots 0 0 0 1 2 2 2
  line L133 (-21.2246, 41.059) -> (-19.927, 42.0848)
  spline S130 degree 2 poles (-22.0427, 40.8539) (-22.1589, 40.8539) (-22.3245, 40.7649) (-22.369, 40.6636) knots 0 0 0 1 2 2 2
  spline S131 degree 2 poles (-22.369, 40.6636) (-22.3987, 40.5919) (-22.416, 40.4164) (-22.416, 40.2854) knots 0 0 0 1 2 2 2
  line L134 (-22.416, 40.2854) -> (-22.416, 40.0284)
  line L135 (-22.416, 40.0284) -> (-21.5954, 40.0284)
  line L136 (-21.5954, 40.0284) -> (-21.5954, 40.2483)
  spline S132 degree 2 poles (-21.5954, 40.2483) (-21.5954, 40.4065) (-21.6349, 40.6314) (-21.6967, 40.7081) knots 0 0 0 1 2 2 2
  spline S133 degree 2 poles (-21.6967, 40.7081) (-21.756, 40.7822) (-21.9142, 40.8539) (-22.0427, 40.8539) knots 0 0 0 1 2 2 2
  line L137 (-19.927, 41.9834) -> (-22.977, 43.0141)
  line L138 (-22.977, 43.0141) -> (-22.977, 43.8495)
  line L139 (-22.977, 43.8495) -> (-19.927, 44.8802)
  line L140 (-19.927, 44.8802) -> (-19.927, 44.0917)
  line L141 (-19.927, 44.0917) -> (-20.5499, 43.9014)
  line L142 (-20.5499, 43.9014) -> (-20.5499, 42.9424)
  line L143 (-20.5499, 42.9424) -> (-19.927, 42.7496)
  line L144 (-19.927, 42.7496) -> (-19.927, 41.9834)
  line L145 (-21.1035, 43.7334) -> (-22.1119, 43.4219)
  line L146 (-22.1119, 43.4219) -> (-21.1035, 43.108)
  line L147 (-21.1035, 43.108) -> (-21.1035, 43.7334)
  spline S134 degree 2 poles (-19.8726, 46.1259) (-19.8726, 45.7749) (-20.0086, 45.246) (-20.1074, 45.0186) knots 0 0 0 1 2 2 2
  line L148 (-20.1074, 45.0186) -> (-20.8341, 45.0186)
  line L149 (-20.8341, 45.0186) -> (-20.8341, 45.0878)
  spline S135 degree 2 poles (-20.8341, 45.0878) (-20.6389, 45.3177) (-20.4288, 45.8688) (-20.4288, 46.1284) knots 0 0 0 1 2 2 2
  spline S136 degree 2 poles (-20.4288, 46.1284) (-20.4288, 46.1951) (-20.4584, 46.4101) (-20.4881, 46.4744) knots 0 0 0 1 2 2 2
  spline S137 degree 2 poles (-20.4881, 46.4744) (-20.5227, 46.5535) (-20.6487, 46.6647) (-20.7501, 46.6647) knots 0 0 0 1 2 2 2
  spline S138 degree 2 poles (-20.7501, 46.6647) (-20.8662, 46.6647) (-21.0096, 46.4843) (-21.0417, 46.3607) knots 0 0 0 1 2 2 2
  spline S139 degree 2 poles (-21.0417, 46.3607) (-21.0837, 46.205) (-21.1554, 45.8515) (-21.2098, 45.6958) knots 0 0 0 1 2 2 2
  spline S140 degree 2 poles (-21.2098, 45.6958) (-21.3334, 45.3424) (-21.756, 45.0359) (-22.0724, 45.0359) knots 0 0 0 1 2 2 2
  spline S141 degree 2 poles (-22.0724, 45.0359) (-22.5, 45.0359) (-23.0314, 45.7601) (-23.0314, 46.3039) knots 0 0 0 1 2 2 2
  spline S142 degree 2 poles (-23.0314, 46.3039) (-23.0314, 46.5757) (-22.9202, 47.1146) (-22.8262, 47.3271) knots 0 0 0 1 2 2 2
  line L150 (-22.8262, 47.3271) -> (-22.1292, 47.3271)
  line L151 (-22.1292, 47.3271) -> (-22.1292, 47.2604)
  spline S143 degree 2 poles (-22.1292, 47.2604) (-22.2751, 47.0898) (-22.4753, 46.6005) (-22.4753, 46.3434) knots 0 0 0 1 2 2 2
  spline S144 degree 2 poles (-22.4753, 46.3434) (-22.4753, 46.2421) (-22.4456, 46.0839) (-22.4061, 45.9949) knots 0 0 0 1 2 2 2
  spline S145 degree 2 poles (-22.4061, 45.9949) (-22.3739, 45.9232) (-22.2454, 45.8194) (-22.1663, 45.8194) knots 0 0 0 1 2 2 2
  spline S146 degree 2 poles (-22.1663, 45.8194) (-22.0477, 45.8194) (-21.9117, 45.985) (-21.8574, 46.2223) knots 0 0 0 1 2 2 2
  spline S147 degree 2 poles (-21.8574, 46.2223) (-21.8228, 46.3755) (-21.756, 46.6598) (-21.6992, 46.8229) knots 0 0 0 1 2 2 2
  spline S148 degree 2 poles (-21.6992, 46.8229) (-21.583, 47.1393) (-21.1974, 47.4482) (-20.8811, 47.4482) knots 0 0 0 1 2 2 2
  spline S149 degree 2 poles (-20.8811, 47.4482) (-20.4263, 47.4482) (-19.8726, 46.7339) (-19.8726, 46.1259) knots 0 0 0 1 2 2 2
  line L152 (-19.927, 47.8412) -> (-22.977, 47.8412)
  line L153 (-22.977, 47.8412) -> (-22.977, 49.9026)
  line L154 (-22.977, 49.9026) -> (-22.3962, 49.9026)
  line L155 (-22.3962, 49.9026) -> (-22.3962, 48.6025)
  line L156 (-22.3962, 48.6025) -> (-21.8598, 48.6025)
  line L157 (-21.8598, 48.6025) -> (-21.8598, 49.8012)
  line L158 (-21.8598, 49.8012) -> (-21.279, 49.8012)
  line L159 (-21.279, 49.8012) -> (-21.279, 48.6025)
  line L160 (-21.279, 48.6025) -> (-20.5079, 48.6025)
  line L161 (-20.5079, 48.6025) -> (-20.5079, 49.9026)
  line L162 (-20.5079, 49.9026) -> (-19.927, 49.9026)
  line L163 (-19.927, 49.9026) -> (-19.927, 47.8412)
  line L164 (-19.927, 53.2393) -> (-19.927, 52.3075)
  line L165 (-19.927, 52.3075) -> (-21.0467, 51.4597)
  line L166 (-21.0467, 51.4597) -> (-21.0467, 51.1829)
  line L167 (-21.0467, 51.1829) -> (-19.927, 51.1829)
  line L168 (-19.927, 51.1829) -> (-19.927, 50.4216)
  line L169 (-19.927, 50.4216) -> (-22.977, 50.4216)
  line L170 (-22.977, 50.4216) -> (-22.977, 51.6475)
  spline S150 degree 2 poles (-22.977, 51.6475) (-22.977, 51.9021) (-22.9128, 52.2778) (-22.8139, 52.4385) knots 0 0 0 1 2 2 2
  spline S151 degree 2 poles (-22.8139, 52.4385) (-22.7101, 52.6016) (-22.3863, 52.7944) (-22.1391, 52.7944) knots 0 0 0 1 2 2 2
  spline S152 degree 2 poles (-22.1391, 52.7944) (-21.7906, 52.7944) (-21.3532, 52.478) (-21.2246, 52.2135) knots 0 0 0 1 2 2 2
  line L171 (-21.2246, 52.2135) -> (-19.927, 53.2393)
  spline S153 degree 2 poles (-22.0427, 52.0084) (-22.1589, 52.0084) (-22.3245, 51.9194) (-22.369, 51.8181) knots 0 0 0 1 2 2 2
  spline S154 degree 2 poles (-22.369, 51.8181) (-22.3987, 51.7464) (-22.416, 51.5709) (-22.416, 51.4399) knots 0 0 0 1 2 2 2
  line L172 (-22.416, 51.4399) -> (-22.416, 51.1829)
  line L173 (-22.416, 51.1829) -> (-21.5954, 51.1829)
  line L174 (-21.5954, 51.1829) -> (-21.5954, 51.4028)
  spline S155 degree 2 poles (-21.5954, 51.4028) (-21.5954, 51.561) (-21.6349, 51.7859) (-21.6967, 51.8626) knots 0 0 0 1 2 2 2
  spline S156 degree 2 poles (-21.6967, 51.8626) (-21.756, 51.9367) (-21.9142, 52.0084) (-22.0427, 52.0084) knots 0 0 0 1 2 2 2
  line L175 (-14.9053, 32.0487) -> (-17.3744, 32.0487)
  line L176 (-17.3744, 32.0487) -> (-17.3744, 31.1465)
  line L177 (-17.3744, 31.1465) -> (-17.9553, 31.1465)
  line L178 (-17.9553, 31.1465) -> (-17.9553, 33.717)
  line L179 (-17.9553, 33.717) -> (-17.3744, 33.717)
  line L180 (-17.3744, 33.717) -> (-17.3744, 32.8149)
  line L181 (-17.3744, 32.8149) -> (-14.9053, 32.8149)
  line L182 (-14.9053, 32.8149) -> (-14.9053, 32.0487)
  line L183 (-14.9053, 37.8323) -> (-14.9053, 37.0661)
  line L184 (-14.9053, 37.0661) -> (-16.2573, 37.0661)
  line L185 (-16.2573, 37.0661) -> (-16.2573, 36.0256)
  line L186 (-16.2573, 36.0256) -> (-14.9053, 36.0256)
  line L187 (-14.9053, 36.0256) -> (-14.9053, 35.2593)
  line L188 (-14.9053, 35.2593) -> (-17.9553, 35.2593)
  line L189 (-17.9553, 35.2593) -> (-17.9553, 36.0256)
  line L190 (-17.9553, 36.0256) -> (-16.8381, 36.0256)
  line L191 (-16.8381, 36.0256) -> (-16.8381, 37.0661)
  line L192 (-16.8381, 37.0661) -> (-17.9553, 37.0661)
  line L193 (-17.9553, 37.0661) -> (-17.9553, 37.8323)
  line L194 (-17.9553, 37.8323) -> (-14.9053, 37.8323)
  spline S157 degree 2 poles (-14.841, 39.6984) (-14.841, 39.083) (-15.4342, 38.4206) (-16.0076, 38.4206) knots 0 0 0 1 2 2 2
  line L195 (-16.0076, 38.4206) -> (-17.9553, 38.4206)
  line L196 (-17.9553, 38.4206) -> (-17.9553, 39.1868)
  line L197 (-17.9553, 39.1868) -> (-16.0521, 39.1868)
  spline S158 degree 2 poles (-16.0521, 39.1868) (-15.7333, 39.1868) (-15.4218, 39.4265) (-15.4218, 39.6984) knots 0 0 0 1 2 2 2
  spline S159 degree 2 poles (-15.4218, 39.6984) (-15.4218, 39.9629) (-15.7209, 40.21) (-16.0521, 40.21) knots 0 0 0 1 2 2 2
  line L198 (-16.0521, 40.21) -> (-17.9553, 40.21)
  line L199 (-17.9553, 40.21) -> (-17.9553, 40.9762)
  line L200 (-17.9553, 40.9762) -> (-16.0101, 40.9762)
  spline S160 degree 2 poles (-16.0101, 40.9762) (-15.4466, 40.9762) (-14.841, 40.3311) (-14.841, 39.6984) knots 0 0 0 1 2 2 2
  line L201 (-14.9053, 43.5986) -> (-14.9053, 41.5645)
  line L202 (-14.9053, 41.5645) -> (-17.9553, 41.5645)
  line L203 (-17.9553, 41.5645) -> (-17.9553, 42.3307)
  line L204 (-17.9553, 42.3307) -> (-15.4861, 42.3307)
  line L205 (-15.4861, 42.3307) -> (-15.4861, 43.5986)
  line L206 (-15.4861, 43.5986) -> (-14.9053, 43.5986)
  spline S161 degree 2 poles (-15.8396, 46.4015) (-15.6122, 46.4015) (-15.2686, 46.2285) (-15.1549, 46.0851) knots 0 0 0 1 2 2 2
  spline S162 degree 2 poles (-15.1549, 46.0851) (-15.019, 45.9121) (-14.9053, 45.5018) (-14.9053, 45.183) knots 0 0 0 1 2 2 2
  line L207 (-14.9053, 45.183) -> (-14.9053, 43.9644)
  line L208 (-14.9053, 43.9644) -> (-17.9553, 43.9644)
  line L209 (-17.9553, 43.9644) -> (-17.9553, 45.0396)
  spline S163 degree 2 poles (-17.9553, 45.0396) (-17.9553, 45.3758) (-17.9034, 45.7218) (-17.8218, 45.8726) knots 0 0 0 1 2 2 2
  spline S164 degree 2 poles (-17.8218, 45.8726) (-17.7353, 46.0382) (-17.4387, 46.1988) (-17.2459, 46.1988) knots 0 0 0 1 2 2 2
  spline S165 degree 2 poles (-17.2459, 46.1988) (-17.0235, 46.1988) (-16.675, 45.9764) (-16.5934, 45.7786) knots 0 0 0 1 2 2 2
  line L210 (-16.5934, 45.7786) -> (-16.5786, 45.7786)
  spline S166 degree 2 poles (-16.5786, 45.7786) (-16.5193, 46.0629) (-16.151, 46.4015) (-15.8396, 46.4015) knots 0 0 0 1 2 2 2
  spline S167 degree 2 poles (-15.8519, 45.6106) (-15.9953, 45.6106) (-16.1559, 45.4969) (-16.1979, 45.3832) knots 0 0 0 1 2 2 2
  spline S168 degree 2 poles (-16.1979, 45.3832) (-16.2251, 45.314) (-16.2301, 45.0693) (-16.2301, 44.8666) knots 0 0 0 1 2 2 2
  line L211 (-16.2301, 44.8666) -> (-16.2301, 44.7257)
  line L212 (-16.2301, 44.7257) -> (-15.4614, 44.7257)
  line L213 (-15.4614, 44.7257) -> (-15.4614, 44.7677)
  spline S169 degree 2 poles (-15.4614, 44.7677) (-15.4614, 45.0643) (-15.4688, 45.2917) (-15.5207, 45.4104) knots 0 0 0 1 2 2 2
  spline S170 degree 2 poles (-15.5207, 45.4104) (-15.5677, 45.5142) (-15.7407, 45.6106) (-15.8519, 45.6106) knots 0 0 0 1 2 2 2
  spline S171 degree 2 poles (-17.0951, 45.4202) (-17.1693, 45.4202) (-17.325, 45.3436) (-17.3596, 45.2645) knots 0 0 0 1 2 2 2
  spline S172 degree 2 poles (-17.3596, 45.2645) (-17.3942, 45.1904) (-17.3992, 44.9828) (-17.3992, 44.7776) knots 0 0 0 1 2 2 2
  line L214 (-17.3992, 44.7776) -> (-17.3992, 44.7257)
  line L215 (-17.3992, 44.7257) -> (-16.7516, 44.7257)
  line L216 (-16.7516, 44.7257) -> (-16.7516, 44.8221)
  spline S173 degree 2 poles (-16.7516, 44.8221) (-16.7516, 45.0174) (-16.759, 45.1756) (-16.7985, 45.2596) knots 0 0 0 1 2 2 2
  spline S174 degree 2 poles (-16.7985, 45.2596) (-16.843, 45.351) (-16.9938, 45.4202) (-17.0951, 45.4202) knots 0 0 0 1 2 2 2
  line L217 (-14.9053, 46.8414) -> (-17.9553, 46.8414)
  line L218 (-17.9553, 46.8414) -> (-17.9553, 48.9028)
  line L219 (-17.9553, 48.9028) -> (-17.3744, 48.9028)
  line L220 (-17.3744, 48.9028) -> (-17.3744, 47.6027)
  line L221 (-17.3744, 47.6027) -> (-16.8381, 47.6027)
  line L222 (-16.8381, 47.6027) -> (-16.8381, 48.8014)
  line L223 (-16.8381, 48.8014) -> (-16.2573, 48.8014)
  line L224 (-16.2573, 48.8014) -> (-16.2573, 47.6027)
  line L225 (-16.2573, 47.6027) -> (-15.4861, 47.6027)
  line L226 (-15.4861, 47.6027) -> (-15.4861, 48.9028)
  line L227 (-15.4861, 48.9028) -> (-14.9053, 48.9028)
  line L228 (-14.9053, 48.9028) -> (-14.9053, 46.8414)
  line L229 (-14.9053, 52.2395) -> (-14.9053, 51.3077)
  line L230 (-14.9053, 51.3077) -> (-16.0249, 50.4599)
  line L231 (-16.0249, 50.4599) -> (-16.0249, 50.1831)
  line L232 (-16.0249, 50.1831) -> (-14.9053, 50.1831)
  line L233 (-14.9053, 50.1831) -> (-14.9053, 49.4218)
  line L234 (-14.9053, 49.4218) -> (-17.9553, 49.4218)
  line L235 (-17.9553, 49.4218) -> (-17.9553, 50.6478)
  spline S175 degree 2 poles (-17.9553, 50.6478) (-17.9553, 50.9023) (-17.891, 51.278) (-17.7921, 51.4387) knots 0 0 0 1 2 2 2
  spline S176 degree 2 poles (-17.7921, 51.4387) (-17.6883, 51.6018) (-17.3646, 51.7946) (-17.1174, 51.7946) knots 0 0 0 1 2 2 2
  spline S177 degree 2 poles (-17.1174, 51.7946) (-16.7689, 51.7946) (-16.3314, 51.4782) (-16.2029, 51.2138) knots 0 0 0 1 2 2 2
  line L236 (-16.2029, 51.2138) -> (-14.9053, 52.2395)
  spline S178 degree 2 poles (-17.021, 51.0086) (-17.1372, 51.0086) (-17.3028, 50.9196) (-17.3473, 50.8183) knots 0 0 0 1 2 2 2
  spline S179 degree 2 poles (-17.3473, 50.8183) (-17.3769, 50.7466) (-17.3942, 50.5711) (-17.3942, 50.4401) knots 0 0 0 1 2 2 2
  line L237 (-17.3942, 50.4401) -> (-17.3942, 50.1831)
  line L238 (-17.3942, 50.1831) -> (-16.5736, 50.1831)
  line L239 (-16.5736, 50.1831) -> (-16.5736, 50.4031)
  spline S180 degree 2 poles (-16.5736, 50.4031) (-16.5736, 50.5612) (-16.6132, 50.7862) (-16.675, 50.8628) knots 0 0 0 1 2 2 2
  spline S181 degree 2 poles (-16.675, 50.8628) (-16.7343, 50.9369) (-16.8925, 51.0086) (-17.021, 51.0086) knots 0 0 0 1 2 2 2
  line L240 (-14.9053, 53.0527) -> (-17.3744, 53.0527)
  line L241 (-17.3744, 53.0527) -> (-17.3744, 52.1505)
  line L242 (-17.3744, 52.1505) -> (-17.9553, 52.1505)
  line L243 (-17.9553, 52.1505) -> (-17.9553, 54.721)
  line L244 (-17.9553, 54.721) -> (-17.3744, 54.721)
  line L245 (-17.3744, 54.721) -> (-17.3744, 53.8189)
  line L246 (-17.3744, 53.8189) -> (-14.9053, 53.8189)
  line L247 (-14.9053, 53.8189) -> (-14.9053, 53.0527)
  line L248 (-9.8835, 34.2002) -> (-9.8835, 33.439)
  line L249 (-9.8835, 33.439) -> (-11.9053, 33.439)
  line L250 (-11.9053, 33.439) -> (-10.6003, 32.8853)
  line L251 (-10.6003, 32.8853) -> (-10.6003, 32.3613)
  line L252 (-10.6003, 32.3613) -> (-11.9053, 31.8077)
  line L253 (-11.9053, 31.8077) -> (-9.8835, 31.8077)
  line L254 (-9.8835, 31.8077) -> (-9.8835, 31.086)
  line L255 (-9.8835, 31.086) -> (-12.9335, 31.086)
  line L256 (-12.9335, 31.086) -> (-12.9335, 31.9684)
  line L257 (-12.9335, 31.9684) -> (-11.4283, 32.6456)
  line L258 (-11.4283, 32.6456) -> (-12.9335, 33.3179)
  line L259 (-12.9335, 33.3179) -> (-12.9335, 34.2002)
  line L260 (-12.9335, 34.2002) -> (-9.8835, 34.2002)
  spline S182 degree 2 poles (-9.8292, 37.0031) (-9.8292, 36.6521) (-9.9651, 36.1232) (-10.064, 35.8958) knots 0 0 0 1 2 2 2
  line L261 (-10.064, 35.8958) -> (-10.7906, 35.8958)
  line L262 (-10.7906, 35.8958) -> (-10.7906, 35.965)
  spline S183 degree 2 poles (-10.7906, 35.965) (-10.5954, 36.1949) (-10.3853, 36.746) (-10.3853, 37.0056) knots 0 0 0 1 2 2 2
  spline S184 degree 2 poles (-10.3853, 37.0056) (-10.3853, 37.0723) (-10.4149, 37.2873) (-10.4446, 37.3516) knots 0 0 0 1 2 2 2
  spline S185 degree 2 poles (-10.4446, 37.3516) (-10.4792, 37.4307) (-10.6052, 37.5419) (-10.7066, 37.5419) knots 0 0 0 1 2 2 2
  spline S186 degree 2 poles (-10.7066, 37.5419) (-10.8228, 37.5419) (-10.9661, 37.3615) (-10.9982, 37.2379) knots 0 0 0 1 2 2 2
  spline S187 degree 2 poles (-10.9982, 37.2379) (-11.0403, 37.0822) (-11.1119, 36.7287) (-11.1663, 36.573) knots 0 0 0 1 2 2 2
  spline S188 degree 2 poles (-11.1663, 36.573) (-11.2899, 36.2196) (-11.7125, 35.9131) (-12.0289, 35.9131) knots 0 0 0 1 2 2 2
  spline S189 degree 2 poles (-12.0289, 35.9131) (-12.4565, 35.9131) (-12.9879, 36.6373) (-12.9879, 37.181) knots 0 0 0 1 2 2 2
  spline S190 degree 2 poles (-12.9879, 37.181) (-12.9879, 37.4529) (-12.8767, 37.9917) (-12.7828, 38.2043) knots 0 0 0 1 2 2 2
  line L263 (-12.7828, 38.2043) -> (-12.0858, 38.2043)
  line L264 (-12.0858, 38.2043) -> (-12.0858, 38.1376)
  spline S191 degree 2 poles (-12.0858, 38.1376) (-12.2316, 37.967) (-12.4318, 37.4776) (-12.4318, 37.2206) knots 0 0 0 1 2 2 2
  spline S192 degree 2 poles (-12.4318, 37.2206) (-12.4318, 37.1193) (-12.4021, 36.9611) (-12.3626, 36.8721) knots 0 0 0 1 2 2 2
  spline S193 degree 2 poles (-12.3626, 36.8721) (-12.3304, 36.8004) (-12.2019, 36.6966) (-12.1228, 36.6966) knots 0 0 0 1 2 2 2
  spline S194 degree 2 poles (-12.1228, 36.6966) (-12.0042, 36.6966) (-11.8683, 36.8622) (-11.8139, 37.0995) knots 0 0 0 1 2 2 2
  spline S195 degree 2 poles (-11.8139, 37.0995) (-11.7793, 37.2527) (-11.7125, 37.537) (-11.6557, 37.7001) knots 0 0 0 1 2 2 2
  spline S196 degree 2 poles (-11.6557, 37.7001) (-11.5395, 38.0165) (-11.154, 38.3254) (-10.8376, 38.3254) knots 0 0 0 1 2 2 2
  spline S197 degree 2 poles (-10.8376, 38.3254) (-10.3828, 38.3254) (-9.8292, 37.6111) (-9.8292, 37.0031) knots 0 0 0 1 2 2 2
  spline S198 degree 2 poles (-9.8242, 40.0333) (-9.8242, 39.3462) (-10.6547, 38.5404) (-11.4061, 38.5404) knots 0 0 0 1 2 2 2
  spline S199 degree 2 poles (-11.4061, 38.5404) (-12.1302, 38.5404) (-12.9928, 39.3487) (-12.9928, 40.0358) knots 0 0 0 1 2 2 2
  spline S200 degree 2 poles (-12.9928, 40.0358) (-12.9928, 40.2162) (-12.9508, 40.5079) (-12.9162, 40.6413) knots 0 0 0 1 2 2 2
  spline S201 degree 2 poles (-12.9162, 40.6413) (-12.8841, 40.7451) (-12.7778, 40.9898) (-12.7383, 41.0665) knots 0 0 0 1 2 2 2
  line L265 (-12.7383, 41.0665) -> (-12.0116, 41.0665)
  line L266 (-12.0116, 41.0665) -> (-12.0116, 40.9898)
  spline S202 degree 2 poles (-12.0116, 40.9898) (-12.061, 40.933) (-12.1995, 40.7649) (-12.2637, 40.6586) knots 0 0 0 1 2 2 2
  spline S203 degree 2 poles (-12.2637, 40.6586) (-12.3304, 40.5524) (-12.4219, 40.2978) (-12.4219, 40.1569) knots 0 0 0 1 2 2 2
  spline S204 degree 2 poles (-12.4219, 40.1569) (-12.4219, 39.9913) (-12.3181, 39.7169) (-12.1871, 39.5909) knots 0 0 0 1 2 2 2
  spline S205 degree 2 poles (-12.1871, 39.5909) (-12.0709, 39.4772) (-11.673, 39.3314) (-11.4036, 39.3314) knots 0 0 0 1 2 2 2
  spline S206 degree 2 poles (-11.4036, 39.3314) (-11.1193, 39.3314) (-10.7313, 39.4821) (-10.6127, 39.6057) knots 0 0 0 1 2 2 2
  spline S207 degree 2 poles (-10.6127, 39.6057) (-10.4965, 39.7244) (-10.3952, 40.016) (-10.3952, 40.1618) knots 0 0 0 1 2 2 2
  spline S208 degree 2 poles (-10.3952, 40.1618) (-10.3952, 40.3126) (-10.4965, 40.587) (-10.5583, 40.6809) knots 0 0 0 1 2 2 2
  spline S209 degree 2 poles (-10.5583, 40.6809) (-10.6201, 40.7847) (-10.7511, 40.9404) (-10.803, 40.9972) knots 0 0 0 1 2 2 2
  line L267 (-10.803, 40.9972) -> (-10.803, 41.0665)
  line L268 (-10.803, 41.0665) -> (-10.0862, 41.0665)
  spline S210 degree 2 poles (-10.0862, 41.0665) (-10.0467, 40.9824) (-9.9478, 40.7624) (-9.9132, 40.6438) knots 0 0 0 1 2 2 2
  spline S211 degree 2 poles (-9.9132, 40.6438) (-9.8687, 40.5005) (-9.8242, 40.2508) (-9.8242, 40.0333) knots 0 0 0 1 2 2 2
  line L269 (-9.8835, 44.0917) -> (-9.8835, 43.3255)
  line L270 (-9.8835, 43.3255) -> (-11.2355, 43.3255)
  line L271 (-11.2355, 43.3255) -> (-11.2355, 42.285)
  line L272 (-11.2355, 42.285) -> (-9.8835, 42.285)
  line L273 (-9.8835, 42.285) -> (-9.8835, 41.5188)
  line L274 (-9.8835, 41.5188) -> (-12.9335, 41.5188)
  line L275 (-12.9335, 41.5188) -> (-12.9335, 42.285)
  line L276 (-12.9335, 42.285) -> (-11.8163, 42.285)
  line L277 (-11.8163, 42.285) -> (-11.8163, 43.3255)
  line L278 (-11.8163, 43.3255) -> (-12.9335, 43.3255)
  line L279 (-12.9335, 43.3255) -> (-12.9335, 44.0917)
  line L280 (-12.9335, 44.0917) -> (-9.8835, 44.0917)
  spline S212 degree 2 poles (-9.8193, 45.9578) (-9.8193, 45.3424) (-10.4125, 44.68) (-10.9859, 44.68) knots 0 0 0 1 2 2 2
  line L281 (-10.9859, 44.68) -> (-12.9335, 44.68)
  line L282 (-12.9335, 44.68) -> (-12.9335, 45.4462)
  line L283 (-12.9335, 45.4462) -> (-11.0304, 45.4462)
  spline S213 degree 2 poles (-11.0304, 45.4462) (-10.7115, 45.4462) (-10.4001, 45.6859) (-10.4001, 45.9578) knots 0 0 0 1 2 2 2
  spline S214 degree 2 poles (-10.4001, 45.9578) (-10.4001, 46.2223) (-10.6992, 46.4695) (-11.0304, 46.4695) knots 0 0 0 1 2 2 2
  line L284 (-11.0304, 46.4695) -> (-12.9335, 46.4695)
  line L285 (-12.9335, 46.4695) -> (-12.9335, 47.2357)
  line L286 (-12.9335, 47.2357) -> (-10.9884, 47.2357)
  spline S215 degree 2 poles (-10.9884, 47.2357) (-10.4248, 47.2357) (-9.8193, 46.5906) (-9.8193, 45.9578) knots 0 0 0 1 2 2 2
  line L287 (-9.8835, 49.8581) -> (-9.8835, 47.8239)
  line L288 (-9.8835, 47.8239) -> (-12.9335, 47.8239)
  line L289 (-12.9335, 47.8239) -> (-12.9335, 48.5901)
  line L290 (-12.9335, 48.5901) -> (-10.4644, 48.5901)
  line L291 (-10.4644, 48.5901) -> (-10.4644, 49.8581)
  line L292 (-10.4644, 49.8581) -> (-9.8835, 49.8581)
  line L293 (-9.8835, 52.436) -> (-9.8835, 50.0187)
  line L294 (-9.8835, 50.0187) -> (-10.4545, 50.0187)
  line L295 (-10.4545, 50.0187) -> (-12.3527, 51.4251)
  line L296 (-12.3527, 51.4251) -> (-12.3527, 50.0929)
  line L297 (-12.3527, 50.0929) -> (-12.9335, 50.0929)
  line L298 (-12.9335, 50.0929) -> (-12.9335, 52.3544)
  line L299 (-12.9335, 52.3544) -> (-12.3527, 52.3544)
  line L300 (-12.3527, 52.3544) -> (-10.4644, 50.953)
  line L301 (-10.4644, 50.953) -> (-10.4644, 52.436)
  line L302 (-10.4644, 52.436) -> (-9.8835, 52.436)
  line L303 (-9.8835, 52.8339) -> (-12.9335, 52.8339)
  line L304 (-12.9335, 52.8339) -> (-12.9335, 54.8953)
  line L305 (-12.9335, 54.8953) -> (-12.3527, 54.8953)
  line L306 (-12.3527, 54.8953) -> (-12.3527, 53.5952)
  line L307 (-12.3527, 53.5952) -> (-11.8163, 53.5952)
  line L308 (-11.8163, 53.5952) -> (-11.8163, 54.7939)
  line L309 (-11.8163, 54.7939) -> (-11.2355, 54.7939)
  line L310 (-11.2355, 54.7939) -> (-11.2355, 53.5952)
  line L311 (-11.2355, 53.5952) -> (-10.4644, 53.5952)
  line L312 (-10.4644, 53.5952) -> (-10.4644, 54.8953)
  line L313 (-10.4644, 54.8953) -> (-9.8835, 54.8953)
  line L314 (-9.8835, 54.8953) -> (-9.8835, 52.8339)
  point P0 (0, 0)
  point P1 (-40, 105.6591)
  constraints: 4 end point, 1 midpoint, 1 perpendicular, 1 point on line, 1 vertical, 2 other
emboss "Emboss1" sketch "Sketch4" operation cut depth 5 direction (1, 0, 0) contours L48 S37 S38 S39 L49 S40 S35 S36 L46 L8 | L8 L46 L47 L48 | L138 L139 L140 L141 L142 L8 L147 L145 L146 | L8 L146 L147 L142 L143 L144 L133 L137 L138 | L137 L126 L127 L128 L129 L130 L131 L132 S127 S128 S129 L133 | L133 L126 L137 | L205 L206 L201 L8 | L8 L201 L202 L203 L204 L205 | L277 L278 L279 L280 L269 L270 L271 L8 | L8 L271 L272 L273 L274 L275 L276 L277 | S0 L9 L10 S1 S2 S3 S4 S5 S6 S7 S8 L11 L12 S9 S10 S11 S12 S13 S14 S15 | L13 L14 L15 L16 L17 L18 L19 L20 L21 L22 L23 L24 | L25 L26 L27 L28 L29 L30 L31 L32 L33 L34 | L35 L36 L37 L38 L39 L40 L41 S16 S17 S18 L42 | S23 S24 S25 S26 | S49 S50 S51 S52 | L56 L57 L58 L59 L60 L61 L62 L63 | L64 L65 L66 L67 L68 L69 L70 L71 L72 L73 L74 L75 | S61 S62 S63 S64 L76 L77 S65 S66 S67 S68 S69 S70 S71 S72 L78 L79 S73 S74 | S75 L80 L81 S76 S77 S78 S79 S80 S81 S82 S83 L82 L83 S84 S85 S86 S87 S88 S89 S90 | L84 L85 S91 S92 S93 S94 S95 L86 L87 S96 S97 S98 S99 L88 L89 | S100 S101 S102 S103 S104 S105 S106 S107 | L90 L91 L92 L93 L94 L95 S112 S113 L96 L97 L98 L99 | S114 S115 S116 L100 L101 S117 S118 S119 S120 S121 S122 S123 L102 L103 L104 L105 L106 L107 S124 S125 S126 | L108 L109 L110 L111 L112 L113 L114 L115 | L116 L117 L118 L119 L120 L121 L122 L123 L124 L125 | S134 L148 L149 S135 S136 S137 S138 S139 S140 S141 S142 L150 L151 S143 S144 S145 S146 S147 S148 S149 | L152 L153 L154 L155 L156 L157 L158 L159 L160 L161 L162 L163 | L164 L165 L166 L167 L168 L169 L170 S150 S151 S152 L171 | L175 L176 L177 L178 L179 L180 L181 L182 | L183 L184 L185 L186 L187 L188 L189 L190 L191 L192 L193 L194 | S157 L195 L196 L197 S158 S159 L198 L199 L200 S160 | S161 S162 L207 L208 L209 S163 S164 S165 L210 S166 | L217 L218 L219 L220 L221 L222 L223 L224 L225 L226 L227 L228 | L229 L230 L231 L232 L233 L234 L235 S175 S176 S177 L236 | L240 L241 L242 L243 L244 L245 L246 L247 | L248 L249 L250 L251 L252 L253 L254 L255 L256 L257 L258 L259 L260 | S182 L261 L262 S183 S184 S185 S186 S187 S188 S189 S190 L263 L264 S191 S192 S193 S194 S195 S196 S197 | S198 S199 S200 S201 L265 L266 S202 S203 S204 S205 S206 S207 S208 S209 L267 L268 S210 S211 | S212 L281 L282 L283 S213 S214 L284 L285 L286 S215 | L287 L288 L289 L290 L291 L292 | L293 L294 L295 L296 L297 L298 L299 L300 L301 L302 | L303 L304 L305 L306 L307 L308 L309 L310 L311 L312 L313 L314
body "Solid2"
